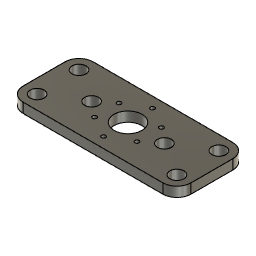
ex38 (Autodesk Fusion 360 design; units mm, degrees)
Autodesk Fusion 360 part; units mm, degrees
sketch "Sketch1" plane through (0, 0, 0) normal (0, 0, 1) x (1, 0, 0)
  line L0 (50, -25) -> (-50, -25)
  line L1 (-60, -15) -> (-60, 15)
  line L2 (-50, 25) -> (50, 25)
  line L3 (60, 15) -> (60, -15)
  arc A0 (60, 15) -> (50, 25) centre (50, 15) ccw
  arc A1 (50, -25) -> (60, -15) centre (50, -15) ccw
  arc A2 (-50, 25) -> (-60, 15) centre (-50, 15) ccw
  arc A3 (-60, -15) -> (-50, -25) centre (-50, -15) ccw
  circle A4 centre (0, 0) radius 10
  circle A5 centre (0, 17.5) radius 1.5
  circle A6 centre (-15.1554, 8.75) radius 1.5
  circle A7 centre (-15.1554, -8.75) radius 1.5
  circle A8 centre (0, -17.5) radius 1.5
  circle A9 centre (15.1554, -8.75) radius 1.5
  circle A10 centre (15.1554, 8.75) radius 1.5
  circle A11 centre (50, 15) radius 5
  circle A12 centre (50, -15) radius 5
  circle A13 centre (-50, -15) radius 5
  circle A14 centre (-50, 15) radius 5
  circle A15 centre (-26, 0) radius 5
  circle A16 centre (26, 0) radius 5
  arc A17 (-14.3505, -10.0157) -> (-1.4986, -17.4357) centre (0, 0) ccw
  arc A18 (1.4986, -17.4357) -> (14.3505, -10.0157) centre (0, 0) ccw
  arc A19 (15.8491, -7.42) -> (15.8491, 7.42) centre (0, 0) ccw
  arc A20 (14.3505, 10.0157) -> (1.4986, 17.4357) centre (0, 0) ccw
  arc A21 (-1.4986, 17.4357) -> (-14.3505, 10.0157) centre (0, 0) ccw
  arc A22 (-15.8491, 7.42) -> (-15.8491, -7.42) centre (0, 0) ccw
  dimension "d3" = 10
  dimension "d4" = 10
  dimension "d5" = 10
  dimension "d6" = 10
  dimension "d7" = 20
  dimension "d8" = 35
  dimension "d9" = 3
  dimension "d11" = 360
  dimension "d12" = 10
  dimension "d13" = 10
  dimension "d14" = 10
  dimension "d15" = 10
  dimension "d16" = 26
  dimension "d17" = 10
  dimension "d18" = 26
  dimension "d19" = 10
  constraint horizontal L0
  constraint perpendicular L0 L1
  constraint parallel L0 L2
  constraint parallel L1 L3
  constraint coincident A4.centre A17.centre
  constraint tangent L3 A0
  constraint tangent L2 A0
  constraint tangent L3 A1
  constraint tangent L0 A1
  constraint tangent L1 A2
  constraint tangent L2 A2
  constraint tangent L1 A3
  constraint tangent L0 A3
  constraint coincident A5.centre A17
  constraint concentric A0 A11
  constraint concentric A1 A12
  constraint concentric A3 A13
  constraint concentric A2 A14
  constraint coincident A7 A22.end
  constraint coincident A7 A17.start
  constraint coincident A8 A17.end
  constraint coincident A8 A18.start
  constraint concentric A17 A18
  constraint coincident A9 A18.end
  constraint coincident A9 A19.start
  constraint concentric A18 A19
  constraint coincident A10 A19.end
  constraint coincident A10 A20.start
  constraint concentric A19 A20
  constraint coincident A5 A20.end
  constraint coincident A5 A21.start
  constraint concentric A20 A21
  constraint coincident A6 A21.end
  constraint coincident A6 A22.start
  constraint concentric A21 A22
  measures "d3" radius of A0
  measures "d4" radius of A1
  measures "d5" radius of A2
  measures "d6" radius of A3
  measures "d7" diameter of A4
  measures "d8" diameter of A17
  measures "d9" diameter of A5
  measures "d12" diameter of A11
  measures "d13" diameter of A12
  measures "d14" diameter of A13
  measures "d15" diameter of A14
  measures "d16" distance of A4.centre A15.centre
  measures "d17" diameter of A15
  measures "d18" distance of A4.centre A16.centre
  measures "d19" diameter of A16
extrude "Extrude1" add sketch "Sketch1" along normal blind 7 contours L0 L1 L2 L3 A0 A1 A2 A3 | A5 A6 A7 A8 A9 A10 A17 A18 A19 A20 A21 A22
